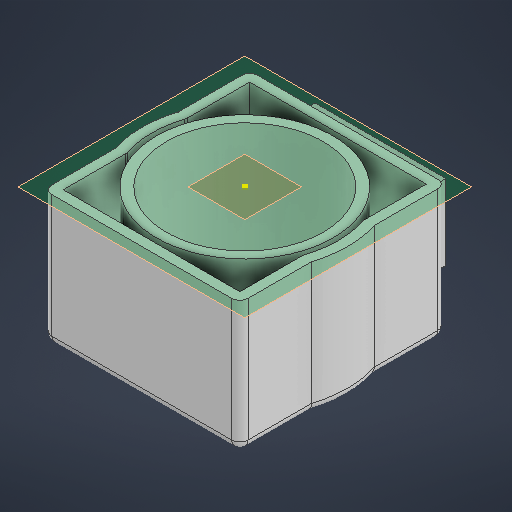
# Autodesk Inventor part: I-bolt compatable floater for in-situ water detection v5
Saved by Autodesk Inventor 2026 (Build 300175050, 175E)
## iProperties
Created: 2025-05-30
Part Number: I-bolt compatable floater for in-situ water detection v5
Material: Generic
Document SubType Name: Modeling
Designer: localuser
Density: 1 g/cm^3
Appearance: Default
Author: localuser
Autodesk Inventor part; units mm, degrees
ref_plane "YZ Plane" through (0, 0, 0) normal (1, 0, 0) x (0, 1, 0)
ref_plane "XZ Plane" through (0, 0, 0) normal (0, 1, 0) x (-1, 0, 0)
ref_plane "XY Plane" through (0, 0, 0) normal (0, 0, 1) x (1, 0, 0)
sketch "Sketch1" plane through (0, 0, 0) normal (0, 1, 0) x (-1, 0, 0)
  circle A0 centre (0, 0) radius 40.005
  dimension "d0" = 80.01
  constraints: 1 centre point, 1 coincident
  measures "d0" diameter of A0
extrude "Extrusion1" add sketch "Sketch1" along normal blind 50.8
ref_plane "Work Plane2" through (0, 50.8, 0) normal (0, 1, 0) x (1, 0, 0)
sketch "Sketch2" plane through (0, 50.8, 0) normal (0, 1, 0) x (1, 0, 0)
  circle A0 centre (0, 0) radius 30.48
  dimension "d5" = 60.96
  constraints: 1 centre point, 1 coincident
  measures "d5" diameter of A0
hole "Hole1" at (0, 50.8, 0) direction (0, -1, 0) diameter 60.96 end through all
ref_plane "Work Plane1" through (0, 50.8, 0) normal (0, 1, 0) x (1, 0, 0)
sketch "Sketch3" plane through (0, 50.8, 0) normal (0, 1, 0) x (1, 0, 0)
  line L0 (0, -31.4608) -> (0, -36.83)
  circle A0 centre (0, 0) radius 36.83 projected
  circle A1 centre (0, 0) radius 30.48 projected
  line L1 (0, -30.48) -> (38.1, -30.48)
  line L2 (38.1, -30.48) -> (38.1, -40.005)
  line L3 (38.1, -40.005) -> (0, -40.005)
  line L4 (0, -40.005) -> (0, -30.48)
  line L5 (0, -40.005) -> (0, -30.48)
  line L6 (0, -30.48) -> (-38.1, -30.48)
  line L7 (-38.1, -30.48) -> (-38.1, -40.005)
  line L8 (-38.1, -40.005) -> (0, -40.005)
  circle A2 centre (0, 0) radius 40.005 projected
  arc A3 (0, -40.005) -> (25.9108, -30.48) centre (0, 0) ccw
  arc A4 (0, -40.005) -> (-25.9108, -30.48) centre (0, 0) ccw
  dimension "d13" = 38.1
  dimension "d14" = 38.1
  constraints: 18 end point, 7 point on circle, 4 parallel, 2 centre point, 2 perpendicular, 2 point on line, 2 vertical alignment, 1 horizontal, 1 tangent, 1 vertical, 2 other
  measures "d13" distance of L2.end L3.end
  measures "d14" distance of L6.end L1.start
extrude "Extrusion2" add sketch "Sketch3" against normal blind 50.8 contours A2 L1 L2 L3 | L8 L7 L6 A2
ref_plane "Work Plane3" through (38.1, 50.8, 40.005) normal (0, -1, 0) x (0, 0, -1)
sketch "Sketch4" plane through (0, 50.8, 0) normal (0, 1, 0) x (1, 0, 0)
  line L0 (-38.1, -40.005) -> (-38.1, -30.48) projected
  line L1 (38.1, 40.005) -> (-38.1, 40.005)
  line L2 (-38.1, 40.005) -> (-38.1, -40.005)
  line L3 (-38.1, -40.005) -> (38.1, -40.005)
  line L4 (38.1, -40.005) -> (38.1, 40.005)
  line L5 (38.1, 40.005) -> (-38.1, -40.005) construction
  line L6 (-38.1, 40.005) -> (38.1, -40.005) construction
  arc A0 (25.9108, -30.48) -> (-25.9108, -30.48) centre (0, 0) ccw projected
  arc A1 (-25.9108, -30.48) -> (-38.1, -12.198) centre (0, 0) ccw
  line L7 (-38.1, -30.48) -> (-25.9108, -30.48) projected
  line L8 (-25.9108, -30.48) -> (-38.1, -30.48)
  line L9 (-38.1, -30.48) -> (-38.1, -12.198)
  line L10 (25.9108, -30.48) -> (38.1, -30.48)
  point P0 (38.1, -12.198)
  point P1 (0, 40.005)
  point P2 (38.1, 12.198)
  point P3 (-38.1, 12.198)
  constraints: 18 end point, 3 equal length, 3 point on circle, 3 point on line, 2 midpoint, 1 centre point, 1 horizontal, 1 perpendicular
extrude "Extrusion3" add sketch "Sketch4" against normal blind 50.8 contours L2 A0 L7 | A0 L4 L10 | L2 L1 A0 | L1 L4 A0
shell "Shell1" thickness 3.81 removed faces 1 at (0, 50.8, -36.83)
fillet "Fillet3" radius 3.175 8 edges at (38.1, 0, -26.1015) (40.005, 0, 0) (38.1, 0, 26.1015) (0, 0, 40.005) (0, 0, -40.005) (-38.1, 0, -26.1015) (-40.005, 0, 0) (-38.1, 0, 26.1015)
fillet "Fillet4" radius 3.175 8 edges at (-37.1701, 0.9299, 39.0751) (-38.1, 26.9875, 40.005) (-37.1701, 0.9299, -39.0751) (-38.1, 26.9875, -40.005) (37.1701, 0.9299, -39.0751) (38.1, 26.9875, -40.005) (37.1701, 0.9299, 39.0751) (38.1, 26.9875, 40.005)
sketch "Sketch6" plane through (0, 50.8, 0) normal (0, 1, 0) x (1, 0, 0)
  point P0 (0, 0)
sketch "Sketch7" plane through (34.925, 50.8, -40.005) normal (0, 0, -1) x (-1, 0, 0)
  line L0 (-5.08, -47.625) -> (-3.175, -47.625) projected
  line L1 (-3.175, -47.625) -> (34.925, -46.99)
  line L2 (0.635, -46.99) -> (69.215, -46.99) projected
  line L3 (69.85, 0) -> (0, 0) projected
  line L4 (34.925, 0) -> (34.925, -26.7586)
  line L5 (34.925, 0) -> (34.925, -25.4)
  line L6 (9.525, -10.8332) -> (60.325, -10.8332)
  line L7 (60.325, -10.8332) -> (60.325, -39.9668)
  line L8 (60.325, -39.9668) -> (9.525, -39.9668)
  line L9 (9.525, -39.9668) -> (9.525, -10.8332)
  line L10 (9.525, -10.8332) -> (60.325, -39.9668) construction
  line L11 (60.325, -10.8332) -> (9.525, -39.9668) construction
  point P0 (34.925, -50.8)
  dimension "d23" = 25.4
  dimension "d24" = 50.8
  constraints: 18 end point, 4 midpoint, 2 parallel, 1 horizontal, 1 perpendicular, 1 point on line, 1 vertical
  measures "d23" distance of L4.start L5.end
  measures "d24" distance of L7.end L8.end
extrude "Extrusion4" add sketch "Sketch7" along normal blind 12.7
sketch "Sketch8" plane through (-25.4, 39.9668, -40.005) normal (0, 1, 0) x (1, 0, 0)
  line L0 (0, 12.7) -> (50.8, 12.7) projected
  line L1 (50.8, 12.7) -> (25.4, 12.7)
  circle A0 centre (25.4, 6.3494) radius 4.0427
  point P0 (25.4, -40.005)
  constraints: 2 end point, 1 centre point, 1 midpoint
hole "Hole2" at (0, 39.9668, -46.3544) direction (0, -1, 0) diameter 5.1054 end through all
body "Solid1"
